wire_clip (Autodesk Fusion 360 design; units mm, degrees)
Autodesk Fusion 360 part; units mm, degrees
sketch "Sketch1" plane through (0, 0, 0) normal (0, 1, 0) x (1, 0, 0)
  line L0 (0, 0) -> (20, 0)
  line L1 (20, 0) -> (20, -13)
  line L2 (20, -13) -> (0, -13)
  line L3 (0, -13) -> (0, 0)
  dimension "d1" = 20
  dimension "d2" = 13
  constraint horizontal L0
  constraint vertical L1
  constraint horizontal L2
  constraint vertical L3
  constraint coincident L0.start L3.end
  measures "d1" distance of L1.end L2.end
  measures "d2" distance of L0.end L1.end
extrude "Extrude1" add sketch "Sketch1" along normal blind 3
sketch "Sketch2" plane through (0, 0, 0) normal (0, -1, 0) x (1, 0, 0)
  line L0 (20, 13) -> (0, 13)
  line L1 (0, 13) -> (0, 0)
  line L2 (0, 0) -> (20, 0)
  line L3 (20, 0) -> (20, 13)
  line L4 (1.5, 11.5) -> (18.5, 11.5)
  line L5 (18.5, 11.5) -> (18.5, 1.5)
  line L6 (18.5, 1.5) -> (1.5, 1.5)
  line L7 (1.5, 1.5) -> (1.5, 11.5)
  dimension "d5" = 1.5
  dimension "d6" = 1.5
  dimension "d7" = 1.5
  dimension "d8" = 1.5
  constraint horizontal L4
  constraint vertical L5
  constraint horizontal L6
  constraint vertical L7
  measures "d5" distance of L1 L7
  measures "d6" distance of L3 L5
  measures "d7" distance of L0 L4
  measures "d8" distance of L2 L6
extrude "Extrude2" cut sketch "Sketch2" against normal blind 0.4 contours L4 L5 L6 L7
sketch "Sketch8" plane through (0, 0, 0) normal (1, 0, 0) x (0, 1, 0)
  arc A0 (7, 0) -> (7, 13) centre (7, 6.5) ccw
  line L0 (-5.9096, 6.5) -> (7, 6.5) construction
  line L1 (0, 13) -> (3, 13)
  line L2 (3, 0) -> (3, 13)
  arc A1 (7, 3) -> (7, 10) centre (7, 6.5) ccw
  line L3 (-1, 6.5) -> (7, 6.5) construction
  line L4 (7, 13) -> (3, 13)
  line L5 (7, 0) -> (3, 0)
  line L6 (7, 3) -> (3, 3)
  line L7 (7, 10) -> (3, 10)
  point P0 (0.5452, 6.5)
  point P1 (3, 6.5)
  dimension "d59" = 6.5
  dimension "d60" = 4
  dimension "d62" = 3
  dimension "d63" = 3
  dimension "d64" = 4
  dimension "d65" = 4
  dimension "d66" = 4
  dimension "d67" = 4
  dimension "d68" = 3.5
  constraint horizontal L0
  constraint midpoint L0 P0
  constraint coincident A0.centre L0.end
  constraint perpendicular L2 L3
  constraint midpoint L2 P1
  constraint midpoint L3 P1
  constraint coincident L1.end L2.end
  constraint coincident L2.start L5.end
  measures "d59" distance of L0 L1
  measures "d60" distance of A0.end L2
  measures "d62" distance of L5 L6
  measures "d63" distance of L4 L7
  measures "d64" distance of L2 A0.centre
  measures "d65" distance of A1.end L7.end
  measures "d66" distance of A1.start L6.end
  measures "d67" distance of A0.start L2.start
  measures "d68" radius of A1
extrude "Extrude6" add sketch "Sketch8" along normal blind 20 contours A0 L2 A1 L4 L5 L6 L7
sketch "Sketch9" plane through (0, 0, 13) normal (0, 0, 1) x (1, 0, 0)
  line L0 (0, 7) -> (0, 3)
  line L1 (0, 3) -> (20, 3)
  line L2 (20, 3) -> (20, 7)
  line L3 (20, 7) -> (0, 7)
  line L4 (4, 7) -> (16, 7)
  line L5 (16, 7) -> (16, 3)
  line L6 (16, 3) -> (4, 3)
  line L7 (4, 3) -> (4, 7)
  line L8 (0, 7) -> (0, 3)
  line L9 (4, 3) -> (8, 3)
  line L10 (8, 3) -> (8, 15)
  line L11 (8, 15) -> (4, 15)
  line L12 (4, 15) -> (4, 3)
  line L13 (16, 3) -> (12, 3)
  line L14 (12, 3) -> (12, 15)
  line L15 (12, 15) -> (16, 15)
  line L16 (16, 15) -> (16, 3)
  dimension "d71" = 4
  dimension "d72" = 4
  dimension "d73" = 4
  dimension "d74" = 4
  dimension "d75" = 12
  dimension "d76" = 12
  constraint horizontal L4
  constraint vertical L5
  constraint horizontal L6
  constraint vertical L7
  constraint coincident L1 L5.end
  constraint coincident L3 L4.start
  constraint horizontal L9
  constraint vertical L10
  constraint horizontal L11
  constraint vertical L12
  constraint horizontal L13
  constraint vertical L14
  constraint horizontal L15
  constraint vertical L16
  measures "d71" distance of L7 L8
  measures "d72" distance of L2 L5
  measures "d73" distance of L14.end L15.end
  measures "d74" distance of L10.end L11.end
  measures "d75" distance of L9.end L10.end
  measures "d76" distance of L13.end L14.end
extrude "Extrude7" cut sketch "Sketch9" against normal blind 19 contours L3 L4 L10 L11 L12 | L1 L3 L4 L6 L7 L9 L10 L12 | L3 L4 L14 L15 L16 | L1 L3 L4 L5 L6 L13 L14 L16
extrude "Extrude8" cut sketch "Sketch9" against normal blind 3 contours L1 L3 L4 L6 L10 L14
sketch "Sketch10" plane through (0, 0, 0) normal (0, 0, -1) x (1, 0, 0)
  line L0 (16, -3) -> (16, -7)
  line L1 (16, -7) -> (20, -7)
  line L2 (20, -7) -> (20, -3)
  line L3 (20, -3) -> (16, -3)
  line L4 (16, -3) -> (20, -3)
  line L5 (20, -3) -> (20, -7)
  line L6 (20, -7) -> (16, -7)
  line L7 (16, -7) -> (16, -3)
  line L8 (0, -3) -> (4, -3)
  line L9 (4, -3) -> (4, -7)
  line L10 (4, -7) -> (0, -7)
  line L11 (0, -7) -> (0, -3)
  constraint horizontal L4
  constraint vertical L5
  constraint horizontal L6
  constraint vertical L7
  constraint coincident L1.end L2.start
  constraint coincident L0.start L3.end
  constraint horizontal L8
  constraint vertical L9
  constraint horizontal L10
  constraint vertical L11
extrude "Extrude9" cut sketch "Sketch10" against normal blind 3
fillet "Fillet2" radius 0.5 6 edges at (10, 7, 13) (10, 7, 10) (18, 7, 3) (18, 7, 0) (2, 7, 3) (2, 7, 0)
extrude "Extrude5" [suppressed]
pattern_linear "R-Pattern1" [suppressed]
ref_plane "WorkPlane1" through (7.5, 11, 5) normal (0, 1, 0) x (0, 0, 1)
sketch "Sketch3" plane through (0, 3, 0) normal (0, 1, 0) x (-1, 0, 0)
  line L0 (0, 10) -> (-15, 10)
  line L1 (-15, 10) -> (-15, 0)
  line L2 (-15, 0) -> (0, 0)
  line L3 (0, 0) -> (0, 10)
  line L4 (-15, 10) -> (-9.5, 10)
  line L5 (-9.5, 10) -> (-9.5, 6.5)
  line L6 (-9.5, 6.5) -> (-15, 6.5)
  line L7 (-15, 6.5) -> (-15, 10)
  line L8 (-15, 0) -> (-9.5, 0)
  line L9 (-9.5, 0) -> (-9.5, 3.5)
  line L10 (-9.5, 3.5) -> (-15, 3.5)
  line L11 (-15, 3.5) -> (-15, 0)
  line L12 (0, 0) -> (-5.5, 0)
  line L13 (-5.5, 0) -> (-5.5, 3.5)
  line L14 (-5.5, 3.5) -> (0, 3.5)
  line L15 (0, 3.5) -> (0, 0)
  line L16 (0, 10) -> (-5.5, 10)
  line L17 (-5.5, 10) -> (-5.5, 6.5)
  line L18 (-5.5, 6.5) -> (0, 6.5)
  line L19 (0, 6.5) -> (0, 10)
  dimension "d12" = 5.5
  dimension "d13" = 3.5
  dimension "d14" = 3.5
  dimension "d15" = 5.5
  dimension "d16" = 5.5
  dimension "d17" = 5.5
  dimension "d18" = 3.5
  dimension "d19" = 3.5
  constraint horizontal L4
  constraint vertical L5
  constraint horizontal L6
  constraint vertical L7
  constraint coincident L0.end L1.start
  constraint horizontal L8
  constraint vertical L9
  constraint horizontal L10
  constraint vertical L11
  constraint coincident L1.end L2.start
  constraint horizontal L12
  constraint vertical L13
  constraint horizontal L14
  constraint vertical L15
  constraint coincident L2.end L3.start
  constraint horizontal L16
  constraint vertical L17
  constraint horizontal L18
  constraint vertical L19
  constraint coincident L0.start L3.end
  measures "d12" distance of L5.end L6.end
  measures "d13" distance of L0.end L6.end
  measures "d14" distance of L1.end L10.end
  measures "d15" distance of L9.end L10.end
  measures "d16" distance of L13.end L14.end
  measures "d17" distance of L17.end L18.end
  measures "d18" distance of L16.end L17.end
  measures "d19" distance of L2.end L14.end
sketch "Sketch4" plane through (7.5, 11, 5) normal (0, 1, 0) x (1, 0, 0)
  line L0 (5, -3.5) -> (-5, -3.5)
  line L1 (-5, -3.5) -> (-5, 3.5)
  line L2 (-5, 3.5) -> (5, 3.5)
  line L3 (5, 3.5) -> (5, -3.5)
  line L4 (7.5, -5) -> (7.5, 5)
  line L5 (-7.5, -5) -> (7.5, -5)
  line L6 (-7.5, 5) -> (-2, 5)
  line L7 (-7.5, 5) -> (-7.5, -5)
  line L8 (0, -3.5) -> (0, 3.5)
  line L9 (-5, 0) -> (5, 0)
  dimension "d20" = 2.5
  dimension "d21" = 1.5
  dimension "d22" = 1.5
  dimension "d23" = 2.5
  constraint horizontal L0
  constraint vertical L1
  constraint horizontal L2
  constraint vertical L3
  constraint midpoint L0 L8.start
  constraint midpoint L2 L8.end
  constraint midpoint L1 L9.start
  constraint midpoint L3 L9.end
  measures "d20" distance of L3 L4
  measures "d21" distance of L0 L5
  measures "d22" distance of L2 L6
  measures "d23" distance of L1 L7
sketch "Sketch5" plane through (0, 0, 0) normal (1, 0, 0) x (0, 1, 0)
  spline S0 degree 5 poles (11, 8.5) (10.8709, 8.7581) (10.6017, 9.2406) (10.1648, 9.863) (9.5185, 10.5016) (8.6214, 11.04) (7.6596, 11.3855) (6.6659, 11.5929) (5.6813, 11.6905) (4.7581, 11.6584) (3.9565, 11.4331) (3.459, 11.0352) (3.1875, 10.5819) (3.0545, 10.2062) (3, 10) knots 0 0 0 0 0 0 0.1 0.2 0.3 0.4 0.5 0.6 0.7 0.8 0.9 1 1 1 1 1 1
  line L0 (3, 5) -> (11, 5)
  spline S1 degree 5 poles (11, 1.5) (10.8709, 1.2419) (10.6017, 0.7594) (10.1648, 0.137) (9.5185, -0.5016) (8.6214, -1.04) (7.6596, -1.3855) (6.6659, -1.5929) (5.6813, -1.6905) (4.7581, -1.6584) (3.9565, -1.4331) (3.459, -1.0352) (3.1875, -0.5819) (3.0545, -0.2062) (3, 0) knots 0 0 0 0 0 0 0.1 0.2 0.3 0.4 0.5 0.6 0.7 0.8 0.9 1 1 1 1 1 1
  line L1 (11.5, 7.5) -> (10.5, 9.5)
  line L2 (3.2545, 10.9631) -> (2.7455, 9.0369)
  line L3 (11.5, 2.5) -> (10.5, 0.5)
  line L4 (3.2545, -0.9631) -> (2.7455, 0.9631)
  point P0 (6.2142, 11.6232)
  point P1 (6.2142, -1.6232)
  constraint horizontal L0
  constraint midpoint S0.start L1
  constraint midpoint S0.end L2
  constraint symmetric S0.start L0 S1.start
  constraint symmetric P0 L0 P1
  constraint symmetric S0.end L0 S1.end
  constraint symmetric L0 L1.start L3.start
  constraint symmetric L0 L1.end L3.end
  constraint symmetric L0 L2.start L4.start
  constraint symmetric L0 L2.end L4.end
sweep "Sweep1" [suppressed]
sweep "Sweep2" [suppressed]
sketch "Sketch6" plane through (0, 11, 0) normal (0, 1, 0) x (-1, 0, 0)
  line L0 (0, 5) -> (0, 8.5)
  line L1 (0, 8.5) -> (-5.5, 8.5)
  line L2 (-5.5, 8.5) -> (-5.5, 5)
  line L3 (-5.5, 5) -> (0, 5)
  line L4 (0, 8.5) -> (-15, 8.5)
  line L5 (-15, 8.5) -> (-15, 1.5)
  line L6 (-15, 1.5) -> (0, 1.5)
  line L7 (0, 1.5) -> (0, 8.5)
  constraint horizontal L4
  constraint vertical L5
  constraint horizontal L6
  constraint vertical L7
  constraint coincident L0.end L1.start
extrude "Extrude3" [suppressed]
chamfer "Chamfer1" [suppressed]
chamfer "Chamfer2" [suppressed]
fillet "Fillet1" [suppressed]
sketch "Sketch7" plane through (0, 0, 0) normal (-1, 0, 0) x (0, -1, 0)
  line L0 (-9.5, 3.0663) -> (-9.5, 6.9337)
  spline S0 degree 5 poles (-3, 6.5) (-3.0545, 6.7062) (-3.1875, 7.0819) (-3.459, 7.5352) (-3.9565, 7.9331) (-4.7581, 8.1584) (-5.6813, 8.1905) (-6.6659, 8.0929) (-7.6596, 7.8855) (-8.4299, 7.6088) (-8.9786, 7.3141) (-9.3284, 7.0698) (-9.4993, 6.9343) (-9.5, 6.9337) knots 0 0 0 0 0 0 0.1 0.2 0.3 0.4 0.5 0.6 0.7 0.8 0.800438 0.800438 0.800438 0.800438 0.800438 0.800438
  line L1 (-3, 6.5) -> (-3, 3.5)
  spline S1 degree 5 poles (-3, 3.5) (-3.0545, 3.2938) (-3.1875, 2.9181) (-3.459, 2.4648) (-3.9565, 2.0669) (-4.7581, 1.8416) (-5.6813, 1.8095) (-6.6659, 1.9071) (-7.6596, 2.1145) (-8.4299, 2.3912) (-8.9786, 2.6859) (-9.3284, 2.9302) (-9.4993, 3.0657) (-9.5, 3.0663) knots 0 0 0 0 0 0 0.1 0.2 0.3 0.4 0.5 0.6 0.7 0.8 0.800438 0.800438 0.800438 0.800438 0.800438 0.800438
  spline S2 degree 3 poles (-10.6939, 0.9459) (-10.7913, 1.1051) (-10.8723, 1.2739) (-10.9987, 1.6253) (-11.0439, 1.807) (-11.0703, 1.9918) knots 0 0 0 0 0.056016 0.056016 0.112032 0.112032 0.112032 0.112032
  spline S3 degree 5 poles (-3, 0) (-3.0545, -0.2062) (-3.1875, -0.5819) (-3.459, -1.0352) (-3.9565, -1.4331) (-4.7581, -1.6584) (-5.6813, -1.6905) (-6.6659, -1.5929) (-7.6596, -1.3855) (-8.6214, -1.04) (-9.4366, -0.5507) (-10.0163, -0.006) (-10.399, 0.4851) (-10.6183, 0.8222) (-10.6939, 0.9459) knots 0 0 0 0 0 0 0.1 0.2 0.3 0.4 0.5 0.6 0.7 0.8 0.9 0.954347 0.954347 0.954347 0.954347 0.954347 0.954347
  line L2 (-3, 0) -> (0, 0)
  line L3 (0, 0) -> (0, 10)
  line L4 (0, 10) -> (-3, 10)
  spline S4 degree 5 poles (-3, 10) (-3.0545, 10.2062) (-3.1875, 10.5819) (-3.459, 11.0352) (-3.9565, 11.4331) (-4.7581, 11.6584) (-5.6813, 11.6905) (-6.6659, 11.5929) (-7.6596, 11.3855) (-8.6214, 11.04) (-9.4366, 10.5507) (-10.0163, 10.006) (-10.399, 9.5149) (-10.6183, 9.1778) (-10.6939, 9.0541) knots 0 0 0 0 0 0 0.1 0.2 0.3 0.4 0.5 0.6 0.7 0.8 0.9 0.954347 0.954347 0.954347 0.954347 0.954347 0.954347
  spline S5 degree 3 poles (-11.0703, 8.0082) (-11.0439, 8.193) (-10.9987, 8.3747) (-10.8723, 8.7261) (-10.7913, 8.8949) (-10.6939, 9.0541) knots 0 0 0 0 0.056016 0.056016 0.112032 0.112032 0.112032 0.112032
  line L5 (-11.0703, 8.0082) -> (-11.4444, 5.3889)
  arc A0 (-11.4444, 5.3889) -> (-11.4444, 4.6111) centre (-8.7221, 5) ccw
  line L6 (-11.4444, 4.6111) -> (-11.0703, 1.9918)
  line L7 (-7.0343, 1.9999) -> (-9.4572, -0.4673)
  line L8 (-12.4962, 0.9146) -> (-9.4572, -0.4673)
  line L9 (-7.9222, 3.0854) -> (-7.0343, 1.9999)
  line L10 (-7.9222, 3.0854) -> (-9.5, 3.0854)
  line L11 (-12.5298, 1.0039) -> (-9.5, 3.0854)
  line L12 (-12.5298, 1.0039) -> (-12.4962, 0.9146)
  constraint coincident S1 L7.start
  constraint coincident S3 L7.end
  constraint coincident L0 L10.end
  constraint perpendicular L0 L10
extrude "Extrude4" [suppressed]
